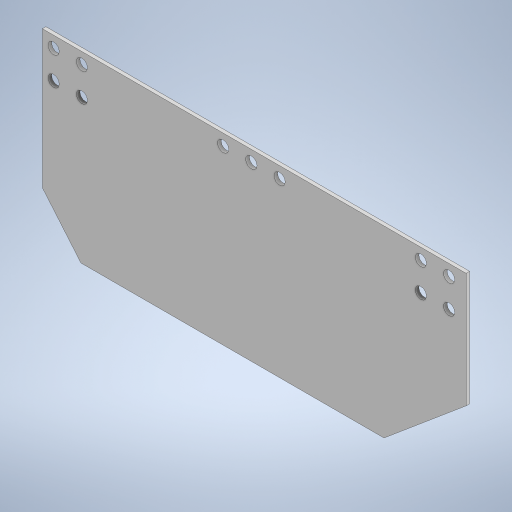
# Autodesk Inventor part: Wing poly tall
Saved by Autodesk Inventor 2023 (Build 270158000, 158)
## iProperties
Created: 2024-01-16
Part Number: Wing poly tall
Material: Generic
Document SubType Name: Modeling
Designer: Robodox
Density: 1 g/cm^3
Appearance: Default
Author: Robodox
Autodesk Inventor part; units mm, degrees
ref_plane "YZ Plane" through (0, 0, 0) normal (1, 0, 0) x (0, 1, 0)
ref_plane "XZ Plane" through (0, 0, 0) normal (0, 1, 0) x (-1, 0, 0)
ref_plane "XY Plane" through (0, 0, 0) normal (0, 0, 1) x (1, 0, 0)
sketch "Sketch1" plane through (0, 0, 0) normal (0, 0, 1) x (1, 0, 0)
  line L0 (-115.6048, 112.2123) -> (74.8952, 112.2123)
  line L1 (74.8952, 112.2123) -> (74.8952, 29.6623)
  line L2 (74.8952, 29.6623) -> (-115.6048, 29.6623)
  line L3 (-115.6048, 29.6623) -> (-115.6048, 112.2123)
  line L4 (74.8952, 70.9373) -> (74.8952, 50.3105)
  line L5 (74.8952, 50.3105) -> (74.8952, 60.6239)
  line L6 (74.8952, 60.6239) -> (37.9963, 29.6623)
  line L7 (74.8952, 50.3105) -> (-115.6048, 50.3105)
  line L8 (-115.6048, 50.3105) -> (-98.2791, 29.6623)
  point P0 (0, 0)
  dimension "d0" = 190.5
  dimension "d1" = 82.55
  constraints: 18 end point, 4 point on line, 2 midpoint, 2 parallel, 2 perpendicular, 1 coincident, 1 horizontal
  measures "d0" distance of L0.start L0.end
  measures "d1" distance of L0.end L1.end
extrude "Extrusion1" add sketch "Sketch1" along normal blind 1.5875 contours L0 L1 L6 L7 L3 | L7 L6 L2 L8
sketch "Sketch2" plane through (0, 0, 1.5875) normal (0, 0, 1) x (1, 0, 0)
  line L0 (-115.6048, 112.2123) -> (-115.6048, 50.3105) projected
  line L1 (-115.6048, 112.2123) -> (-115.6048, 107.142)
  line L2 (-115.6048, 107.142) -> (-110.5257, 107.142)
  circle A0 centre (-110.5257, 107.142) radius 2.54
  line L3 (-110.5257, 107.142) -> (-110.5257, 94.442)
  circle A1 centre (-110.5257, 94.442) radius 2.54
  line L4 (-110.5257, 107.142) -> (-97.8257, 107.142)
  line L5 (-97.8257, 107.142) -> (-97.8257, 94.442)
  circle A2 centre (-97.8257, 107.142) radius 2.54
  circle A3 centre (-97.8257, 94.442) radius 2.54
  line L6 (-97.8257, 107.142) -> (67.2743, 107.142)
  circle A4 centre (67.2743, 107.142) radius 2.54
  line L7 (67.2743, 107.142) -> (67.2743, 94.442)
  line L8 (67.2743, 94.442) -> (54.5743, 94.442)
  line L9 (54.5743, 94.442) -> (54.5743, 107.142)
  circle A5 centre (54.5743, 107.142) radius 2.54
  circle A6 centre (54.5743, 94.442) radius 2.54
  circle A7 centre (67.2743, 94.442) radius 2.54
  line L10 (-97.8257, 107.142) -> (-21.6257, 107.142)
  circle A8 centre (-21.6257, 107.142) radius 2.54
  line L11 (-21.6257, 107.142) -> (-34.3257, 107.142)
  circle A9 centre (-34.3257, 107.142) radius 2.54
  line L12 (-21.6257, 107.142) -> (-8.9257, 107.142)
  circle A10 centre (-8.9257, 107.142) radius 2.54
  point P0 (0, 0)
  dimension "d4" = 5.08
  dimension "d5" = 12.7
  dimension "d6" = 5.08
  dimension "d7" = 12.7
  dimension "d8" = 5.08
  dimension "d9" = 5.08
  dimension "d10" = 165.1
  dimension "d11" = 5.08
  dimension "d12" = 12.7
  dimension "d13" = 12.7
  dimension "d14" = 5.08
  dimension "d15" = 5.08
  dimension "d16" = 5.08
  dimension "d17" = 76.2
  dimension "d18" = 5.08
  dimension "d19" = 12.7
  dimension "d20" = 5.08
  dimension "d21" = 12.7
  dimension "d22" = 5.08
  constraints: 24 end point, 11 centre point, 11 coincident, 5 point on line, 4 horizontal, 3 vertical, 1 perpendicular
  measures "d4" diameter of A0
  measures "d5" distance of L3.start L3.end
  measures "d6" diameter of A1
  measures "d7" distance of L3.start L4.end
  measures "d8" diameter of A2
  measures "d9" diameter of A3
  measures "d10" distance of L6.start L6.end
  measures "d11" diameter of A4
  measures "d12" distance of L7.start L7.end
  measures "d13" distance of L7.end L8.end
  measures "d14" diameter of A5
  measures "d15" diameter of A6
  measures "d16" diameter of A7
  measures "d17" distance of L6.start L10.end
  measures "d18" diameter of A8
  measures "d19" distance of L11.start L11.end
  measures "d20" diameter of A9
  measures "d21" distance of L11.start L12.end
  measures "d22" diameter of A10
extrude "Extrusion2" cut sketch "Sketch2" against normal through all contours A0 L4 L2 | A5 L6 | L6 L9 A5 | A10 L6 | L6 A10 | A8 L6 | L6 A8 | A9 L6 | L6 A9 | A3 | A2 L6 L4 | L4 L5 A2 | A1 | L2 L3 A0 | L4 A0 L3 | L6 A2 L5 | L6 A5 L9 | A4 L7 L6 | L6 L7 A4 | A6 L8 L9 | L9 L8 A6 | A7 L8 L7 | L7 L8 A7
body "Solid1"
